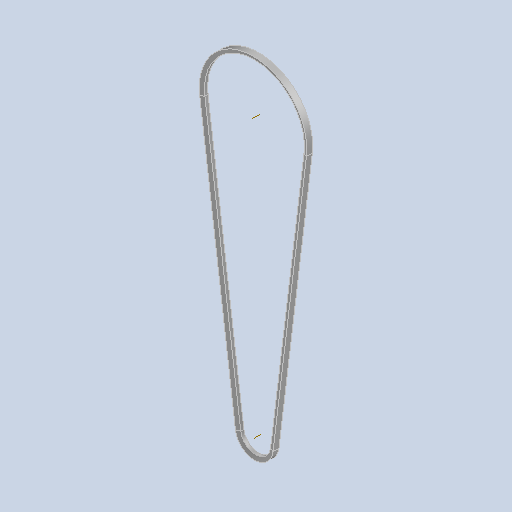
# Autodesk Inventor part: V-Belt
Saved by Autodesk Inventor 2025 (Build 290162000, 162)
## iProperties
Created: 2025-05-25
Part Number: V-Belt
Material: Rubber
Document SubType Name: Modeling
Designer: Abdullah
Density: 0.93 g/cm^3
Appearance: Rubber - Black - Version 1.1
CustomPartVersion: 1
Author: Abdullah
Autodesk Inventor part; units mm, degrees
ref_plane "YZ Plane" through (0, 0, 0) normal (1, 0, 0) x (0, 1, 0)
ref_plane "XZ Plane" through (0, 0, 0) normal (0, 1, 0) x (-1, 0, 0)
sketch "Sketch Path" plane through (0, 0, 0) normal (0, 0, 1) x (1, 0, 0)
  arc A0 (-49.5725, -13.0241) -> (49.6274, -12.5923) centre (0, -6.5) ccw
  arc A1 (145.4323, 767.823) -> (-152.1676, 766.5276) centre (-3.45, 786.1) ccw
  line L0 (145.4323, 767.823) -> (49.6274, -12.5923)
  line L1 (-49.5725, -13.0241) -> (-152.1676, 766.5276)
  constraints: 4 end point, 4 point on circle, 2 centre point
ref_plane "Cross Section Plane" through (49.6274, -12.5923, 0) normal (0.1218, 0.9925, 0) x (0, 0, 1)
sketch "Cross Section" plane through (49.6274, -12.5923, 0) normal (0.1218, 0.9925, 0) x (0, 0, 1)
  line L0 (0, 4.1563) -> (0, -6.8437) construction
  line L1 (-7, 0) -> (7, 0) construction
  line L2 (-8.5128, 4.1563) -> (8.5128, 4.1563)
  line L3 (8.5128, 4.1563) -> (4.5091, -6.8437)
  line L4 (4.5091, -6.8437) -> (-4.5091, -6.8437)
  line L5 (-4.5091, -6.8437) -> (-8.5128, 4.1563)
  point P0 (0, 0)
  point P1 (0, 0)
  point P2 (0, 0)
  dimension "d0" = 14
  dimension "d1" = 4.1563
  dimension "d2" = 40
  dimension "d3" = 11
  constraints: 12 end point, 3 midpoint, 2 parallel, 2 point on line, 1 coincident, 1 perpendicular, 1 vertical, 1 other
  measures "d0" distance of L1.start L1.end
  measures "d1" distance between parallel lines of L2 L1
  measures "d2" angle of L5 L3
  measures "d3" distance between parallel lines of L4 L2
sweep "Belt" add profiles "Cross Section" path "Sketch Path"
equation "\"d0\" = da_Bw"
equation "\"d1\" = da_Hw"
equation "\"d2\" = da_Alfa"
equation "\"d3\" = da_H"
equation "\"da_Alfa\" = 40deg"
equation "\"da_H\" = 11"
equation "\"da_Bw\" = 14"
equation "\"da_Hw\" = 4.15634"
body "Solid1"
